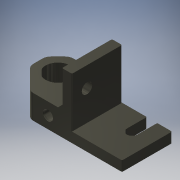
# Autodesk Inventor part: Z Axis Linear Rail Bracket - Left 1.0
Saved by Autodesk Inventor 2016 (Build 200138000, 138)
## iProperties
Created: 2017-02-13
Part Number: Z Axis Linear Rail Bracket - Left 1.0
Material: PC/ABS Plastic
Document SubType Name: Modeling
Designer: Scott
Density: 0.357273 g/cm^3
Appearance: Gunmetal
Author: Scott
Autodesk Inventor part; units mm, degrees
ref_plane "YZ Plane" through (0, 0, 0) normal (1, 0, 0) x (0, 1, 0)
ref_plane "XZ Plane" through (0, 0, 0) normal (0, 1, 0) x (-1, 0, 0)
ref_plane "XY Plane" through (0, 0, 0) normal (0, 0, 1) x (1, 0, 0)
sketch "Sketch1" plane through (0, 0, 0) normal (0, 0, 1) x (1, 0, 0)
  circle A0 centre (0, 0) radius 6.2
  line L0 (0, 0) -> (83.2978, 0) construction
  circle A1 centre (37, 0) radius 2.6
  line L1 (-10, 10) -> (47, 10)
  line L2 (47, 10) -> (47, -15)
  line L3 (47, -15) -> (-10, -15)
  line L4 (-10, -15) -> (-10, 10)
  line L5 (22, 29.5766) -> (22, -18.8569) construction
  dimension "d0" = 12.4
  dimension "d1" = 5.2
  dimension "d2" = 37
  dimension "d3" = 10
  dimension "d4" = 15
  dimension "d5" = 10
  dimension "d6" = 22
  dimension "d7" = 25
  constraints: 12 end point, 3 perpendicular, 2 centre point, 2 horizontal, 1 coincident, 1 point on line, 1 vertical
  measures "d0" diameter of A0
  measures "d1" diameter of A1
  measures "d2" distance of A1.centre L0.start
  measures "d3" distance between parallel lines of L0 L1
  measures "d4" distance between parallel lines of L0 L3
  measures "d5" distance from line of L4 L0.start
  measures "d6" distance from line of L0.start L5
  measures "d7" distance between parallel lines of L2 L5
extrude "Extrusion1" add sketch "Sketch1" along normal blind 5
sketch "Sketch2" plane through (0, 0, 5) normal (0, 0, 1) x (1, 0, 0)
  circle A0 centre (0, 0) radius 6.2 projected
  circle A1 centre (37, 0) radius 2.6 projected
  line L0 (47, 10) -> (-10, 10) projected
  line L1 (-10, 10) -> (-10, -15) projected
  line L2 (-10, -15) -> (47, -15) projected
  line L3 (47, -15) -> (47, 10) projected
  line L4 (22, 10) -> (22, -15)
  dimension "d10" = 22
  constraints: 2 end point, 2 point on line, 1 perpendicular
  measures "d10" distance from line of L4 A0.centre
extrude "Extrusion2" add sketch "Sketch2" along normal blind 7 contours L4 L2 L1 L0
sketch "Sketch3" plane through (0, 0, 12) normal (0, 0, 1) x (1, 0, 0)
  point P0 (0, 0)
sketch "Sketch4" plane through (0, 0, 5) normal (0, 0, 1) x (1, 0, 0)
  circle A0 centre (0, 0) radius 6.2 projected
  line L0 (-10, 10) -> (-10, -15) projected
  line L1 (-10, -15) -> (22, -15) projected
  line L2 (22, -15) -> (22, 10) projected
  line L3 (22, 10) -> (-10, 10) projected
  line L4 (22, 10) -> (17, 10)
  line L5 (17, 10) -> (17, -15)
  line L6 (17, -15) -> (22, -15)
  line L7 (22, -15) -> (22, 10)
  dimension "d13" = 5
  constraints: 8 end point, 2 parallel, 1 horizontal, 1 perpendicular, 1 point on line
  measures "d13" distance between parallel lines of L5 L2
extrude "Extrusion3" add sketch "Sketch4" along normal blind 25 contours L3 L2 L1 L5
chamfer "Chamfer1" distance 6 angle 45 1 edges at (-10, 10, 6)
chamfer "Chamfer2" distance 2 angle 45 1 edges at (17, -2.5, 12)
chamfer "Chamfer3" distance 11 angle 45 1 edges at (-10, -15, 6)
sketch "Sketch5" plane through (22, -15, 5) normal (1, 0, 0) x (0, 0, -1)
  line L0 (0, 25) -> (0, 0) construction
  line L1 (-9, 0) -> (-25, 0) projected
  point P0 (5, 15)
  point P1 (-15, 7.5)
  dimension "d22" = 15
  dimension "d62" = 7.5
  measures "d22" distance from line of point (-15, 7.5) L0
  measures "d62" distance from line of L1 point (-15, 7.5)
hole "Hole1" at (22, -7.5, 20) direction (-1, 0, 0) diameter 5.2 end through all
sketch "Sketch6" plane through (0, 0, 5) normal (0, 0, 1) x (1, 0, 0)
  line L0 (22, 10) -> (22, -15) projected
  line L1 (22, -15) -> (47, -15) projected
  line L2 (47, -15) -> (47, 10) projected
  line L3 (47, 10) -> (22, 10) projected
  circle A0 centre (37, 0) radius 2.6 projected
  line L4 (39.6, 0) -> (39.6, 10)
  circle A1 centre (37, 0) radius 2.6 projected
  line L5 (34.4, 0) -> (34.4, 10)
  line L6 (-4, 10) -> (47, 10) projected
  circle A2 centre (37, 0) radius 2.6 projected
  point P0 (0, 0)
  constraints: 4 end point, 2 point on circle, 2 point on line, 2 vertical, 1 horizontal alignment, 1 parallel, 1 tangent, 1 other
extrude "Extrusion4" cut sketch "Sketch6" against normal through all contours L3 L4 A0 L5
sketch "Sketch7" plane through (0, 0, 12) normal (0, 0, 1) x (1, 0, 0)
  line L0 (15, 10) -> (15, -15) projected
  line L1 (15, 10) -> (-4, 10) projected
  line L2 (-10, 4) -> (-4, 10) projected
  line L3 (-10, 4) -> (-10, -4) projected
  line L4 (1, -15) -> (15, -15) projected
  circle A0 centre (0, 0) radius 6.2 projected
  line L5 (14.25, 10) -> (14.25, 4.25)
  line L6 (14.25, 4.25) -> (4.5141, 4.25)
  line L7 (5.1176, 3.5) -> (15, 3.5)
  line L8 (1, -15) -> (-10, -4) projected
  dimension "d33" = 0.75
  dimension "d34" = 0.75
  dimension "d35" = 3.5
  constraints: 6 end point, 2 point on circle, 2 point on line, 1 horizontal, 1 perpendicular, 1 vertical
  measures "d33" distance between parallel lines of L0 L5
  measures "d34" distance between parallel lines of L6 L7
  measures "d35" distance from line of point (0, 0) L7
extrude "Extrusion5" cut sketch "Sketch7" against normal through all contours L0 L7 A0 L6 L5 L1
fillet "Fillet1" radius 0.5 1 edges at (5.1176, 3.5, 6)
fillet "Fillet2" radius 0.5 1 edges at (4.5141, 4.25, 6)
sketch "Sketch8" plane through (-4, 10, 12) normal (0, 1, 0) x (1, 0, 0)
  line L0 (18.25, 0) -> (18.25, 12) projected
  line L1 (0, 12) -> (18.25, 12) projected
  line L2 (0, 0) -> (0, 12) projected
  line L3 (18.25, 0) -> (0, 0) projected
  point P0 (4, 12)
  point P1 (14, 6)
  dimension "d40" = 10
  dimension "d41" = 6
  measures "d40" horizontal distance of point (4, 12) point (14, 6)
  measures "d41" distance from line of L1 point (14, 6)
hole "Hole2" at (10, 10, 6) direction (0, -1, 0) diameter 3.5 end through all
sketch "Sketch9" plane through (47, -15, 0) normal (0, -1, 0) x (1, 0, 0)
  circle A0 centre (-37, 6) radius 1.75 projected
  circle A1 centre (-37, 6) radius 1.75 projected
  point P0 (-47, 0)
  point P1 (-37, 6)
  constraints: 1 coincident
hole "Hole3" at (10, -15, 6) direction (0, 1, 0) diameter 4.7 depth 5 counterbore diameter 5 counterbore depth 0.5
fillet "Fillet4" radius 0.5 8 edges at (34.4, 10, 2.5) (39.6, 10, 2.5) (47, 10, 2.5) (47, -15, 2.5) (22, 10, 17.5) (17, 10, 22) (22, -15, 17.5) (17, -15, 22)
fillet "Fillet5" radius 4 4 edges at (-4, 10, 6) (-10, 4, 6) (-10, -4, 6) (1, -15, 6)
body "Solid1"
